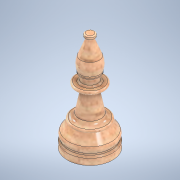
# Autodesk Inventor part: goniec
Saved by Autodesk Inventor 2021 (Build 250183000, 183)
## iProperties
Created: 2021-01-07
Part Number: goniec
Material: Drewno (brzoza)
Document SubType Name: Modeling
Designer: Adam
Density: 0.55 g/cm^3
Appearance: Brzoza — naturalna — polerowana
Author: Adam
Autodesk Inventor part; units mm, degrees
ref_plane "YZ Plane" through (0, 0, 0) normal (1, 0, 0) x (0, 1, 0)
ref_plane "XZ Plane" through (0, 0, 0) normal (0, 1, 0) x (-1, 0, 0)
ref_plane "XY Plane" through (0, 0, 0) normal (0, 0, 1) x (1, 0, 0)
sketch "Szkic1" plane through (0, 0, 0) normal (1, 0, 0) x (0, 1, 0)
  line L0 (0, 0) -> (63.7111, 0)
  line L1 (0, 0) -> (0, -14.5)
  line L2 (0, -14.5) -> (5, -14.5)
  line L3 (5, -14.5) -> (5, -13.5)
  line L4 (5, -13.5) -> (6, -13.5)
  line L5 (6, -13.5) -> (6, -14.5)
  line L6 (6, -14.5) -> (9, -14.5)
  line L7 (9, -14.5) -> (15, -10)
  line L8 (15, -10) -> (15, -11)
  line L9 (15, -11) -> (17, -11)
  line L10 (17, -11) -> (17, -10)
  line L11 (17, 0) -> (35, 0)
  line L12 (35, -4) -> (35, -9)
  line L13 (35, -9) -> (37, -9)
  line L14 (37, -9) -> (37, -6)
  line L15 (37, -6) -> (38, -6)
  line L16 (38, -6) -> (38, -5)
  line L17 (38, -5) -> (41, -5)
  line L18 (41, -5) -> (41, -6)
  line L19 (41, -6) -> (43, -6)
  line L20 (63.7111, 0) -> (63.7111, -3)
  line L21 (63.7111, -3) -> (61.2253, -3)
  line L22 (63.7111, 0) -> (55.5, 0)
  line L23 (51.2612, -5.8204) -> (61.2253, -1.8348)
  line L24 (61.2253, -3) -> (61.2253, -1.8348)
  arc A0 (18.7285, -7.2036) -> (17, -10) centre (20.1262, -10) ccw
  line L25 (18.7285, -7.2036) -> (35, -4)
  arc A1 (43, -6) -> (51.2612, -5.8204) centre (46.8911, 5.1048) ccw
  constraints: 52 end point, 11 perpendicular, 5 vertical, 4 horizontal, 4 point on circle, 4 point on line, 2 centre point, 2 tangent
revolve "Obrót2" add sketch "Szkic1" angle 360 about axis through (0, 0, 0) along (0, 1, 0)
fillet "Zaokrąglenie10" radius 1 1 edges at (0, 5, 14.5)
fillet "Zaokrąglenie11" radius 3 2 edges at (0, 6, 14.5) (0, 9, 14.5)
fillet "Zaokrąglenie12" radius 1 2 edges at (0, 15, 11) (0, 17, 11)
fillet "Zaokrąglenie13" radius 1 2 edges at (0, 35, 9) (0, 37, 9)
fillet "Zaokrąglenie14" radius 3 1 edges at (0, 18.7285, 7.2036)
fillet "Zaokrąglenie15" radius 1 1 edges at (0, 38, 6)
fillet "Zaokrąglenie16" radius 1 1 edges at (0, 41, 6)
fillet "Zaokrąglenie17" radius 3 1 edges at (0, 43, 6)
fillet "Zaokrąglenie18" radius 0.75 2 edges at (0, 61.2253, 3) (0, 63.7111, 3)
